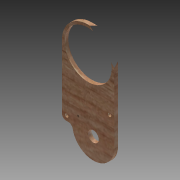
# Autodesk Inventor part: p1
Saved by Autodesk Inventor 2015 (Build 190159000, 159)
## iProperties
Created: 2016-02-03
Part Number: p1
Material: Generic
Document SubType Name: Modeling
Designer: david
Density: 1 g/cm^3
Appearance: Birch - Natural Polished
Author: david
Autodesk Inventor part; units mm, degrees
ref_plane "YZ Plane" through (0, 0, 0) normal (1, 0, 0) x (0, 1, 0)
ref_plane "XZ Plane" through (0, 0, 0) normal (0, 1, 0) x (-1, 0, 0)
ref_plane "XY Plane" through (0, 0, 0) normal (0, 0, 1) x (1, 0, 0)
sketch "Sketch1" plane through (0, 0, 0) normal (0, 1, 0) x (-1, 0, 0)
  line L0 (20, 45) -> (-20, 45)
  line L1 (-20, 45) -> (-20, -45)
  line L2 (-20, -45) -> (20, -45)
  line L3 (20, -45) -> (20, 45)
  line L4 (20, 45) -> (-20, -45) construction
  line L5 (-20, 45) -> (20, -45) construction
  arc A0 (-20, -45) -> (20, -45) centre (0, -45) ccw
  line L6 (20, -45) -> (30, -45)
  line L7 (30, -45) -> (30, 45)
  line L8 (30, 45) -> (20, 45)
  line L9 (20, 45) -> (20, -45)
  point P0 (0, 0)
  dimension "d0" = 40
  dimension "d1" = 90
  dimension "d7" = 10
  dimension "d8" = 90
  constraints: 20 end point, 4 parallel, 3 midpoint, 2 horizontal, 2 perpendicular, 2 point on circle, 1 centre point
  measures "d0" distance of L2.end L1.end
  measures "d1" distance of L1.end L0.end
  measures "d7" distance of L8.end L7.end
  measures "d8" distance of L7.end L6.end
extrude "Extrusion1" add sketch "Sketch1" along normal blind 3.6
sketch "Sketch2" plane through (0, 3.6, 0) normal (0, 1, 0) x (1, 0, 0)
  arc A0 (20, 45) -> (-20, 45) centre (0, 45) ccw projected
  circle A1 centre (0, 45) radius 5.15
  point P0 (0, 0)
  dimension "d4" = 10.3
  constraints: 1 centre point, 1 coincident
  measures "d4" diameter of A1
extrude "Extrusion2" cut sketch "Sketch2" against normal blind 3.6
fillet "Fillet1" radius 4 3 edges at (-20, 1.8, -45) (-30, 1.8, -45) (20, 1.8, 45)
sketch "Sketch3" plane through (0, 0, 0) normal (0, -1, 0) x (1, 0, 0)
  circle A0 centre (-5, 20) radius 22.5
  line L0 (20, 41) -> (20, -45) projected
  line L1 (-30, 45) -> (16, 45) projected
  point P0 (0, 0)
  point P1 (-26, 45)
  dimension "d10" = 45
  dimension "d11" = 25
  dimension "d12" = 25
  constraints: 1 centre point
  measures "d10" diameter of A0
  measures "d11" distance from line of L0 A0.centre
  measures "d12" distance from line of L1 A0.centre
extrude "Extrusion3" cut sketch "Sketch3" against normal blind 10
sketch "Sketch4" plane through (0, 0, 0) normal (0, -1, 0) x (1, 0, 0)
  circle A0 centre (15.5, 40.5) radius 1.625
  circle A1 centre (-25.5, -40.5) radius 1.625
  circle A2 centre (15.5, -19.5) radius 1.625
  line L0 (-30, -41) -> (-30, 45) projected
  line L1 (-23.6643, -45) -> (-26, -45) projected
  line L2 (20, 41) -> (20, -45) projected
  line L3 (-30, 45) -> (16, 45) projected
  point P0 (0, 0)
  point P1 (-30, 41)
  point P2 (-26, 45)
  dimension "d15" = 3.25
  dimension "d17" = 3.25
  dimension "d18" = 3.25
  dimension "d19" = 4.5
  dimension "d20" = 4.5
  dimension "d21" = 4.5
  dimension "d23" = 4.5
  dimension "d24" = 4.5
  dimension "d27" = 60
  constraints: 3 centre point
  measures "d15" diameter of A0
  measures "d17" diameter of A1
  measures "d18" diameter of A2
  measures "d19" distance from line of L0 A1.centre
  measures "d20" distance from line of A1.centre L1
  measures "d21" distance from line of L2 A2.centre
  measures "d23" distance from line of L2 A0.centre
  measures "d24" distance from line of L3 A0.centre
  measures "d27" distance between centres of A0 A2
extrude "Extrusion4" cut sketch "Sketch4" against normal blind 10
fillet "Fillet2" radius 25 1 edges at (-30, 1.8, 45)
body "Solid1"
